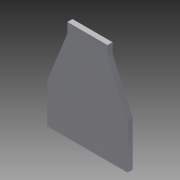
# Autodesk Inventor part: that thing mount
Saved by Autodesk Inventor 2013 (Build 170138000, 138)
## iProperties
Created: 2013-02-04
Part Number: that thing mount
Material: Aluminum 6061
Document SubType Name: Modeling
Designer: Arpan
Density: 1 g/cm^3
Author: Arpan
Autodesk Inventor part; units mm, degrees
ref_plane "YZ Plane" through (0, 0, 0) normal (1, 0, 0) x (0, 1, 0)
ref_plane "XZ Plane" through (0, 0, 0) normal (0, 1, 0) x (-1, 0, 0)
ref_plane "XY Plane" through (0, 0, 0) normal (0, 0, 1) x (1, 0, 0)
sketch "Sketch1" plane through (0, 0, 0) normal (0, 0, 1) x (1, 0, 0)
  line L0 (0, 0) -> (-50.8, 0)
  line L1 (-50.8, 0) -> (-50.8, 57.15)
  line L2 (-50.8, 57.15) -> (0, 57.15)
  line L3 (0, 57.15) -> (0, 0)
  line L4 (-50.8, 0) -> (-50.8, 25.4)
  line L5 (0, 0) -> (0, 25.4)
  line L6 (-25.4, 57.15) -> (-38.1, 57.15)
  line L7 (-25.4, 57.15) -> (-12.7, 57.15)
  line L8 (-12.7, 57.15) -> (0, 28.575)
  line L9 (-38.1, 57.15) -> (-50.8, 25.4)
  dimension "d0" = 50.8
  dimension "d1" = 57.15
  dimension "d2" = 25.4
  dimension "d3" = 12.7
  dimension "d4" = 12.7
  constraints: 20 end point, 4 point on line, 2 midpoint, 2 parallel, 1 horizontal, 1 perpendicular
  measures "d0" distance of L0.start L0.end
  measures "d1" distance of L0.end L1.end
  measures "d2" distance of L0.end L4.end
  measures "d3" distance of L6.start L6.end
  measures "d4" distance of L6.start L7.end
extrude "Extrusion1" add sketch "Sketch1" along normal blind 3.175 contours L0 L1 L9 L2 L8 L3
sketch "Sketch2" plane through (0, 0, 3.175) normal (0, 0, 1) x (1, 0, 0)
  line L0 (-12.7, 57.15) -> (-38.1, 57.15) projected
  line L1 (-50.8, 0) -> (0, 0) projected
  line L2 (-38.1, 57.15) -> (-38.1, 63.5)
  line L3 (-38.1, 63.5) -> (-12.7, 63.5)
  line L4 (-12.7, 63.5) -> (-12.7, 57.15)
  dimension "d7" = 6.35
  constraints: 6 end point, 2 perpendicular, 1 parallel
  measures "d7" distance of L0.end L2.end
extrude "Extrusion2" add sketch "Sketch2" against normal blind 3.175
body "Solid1"
